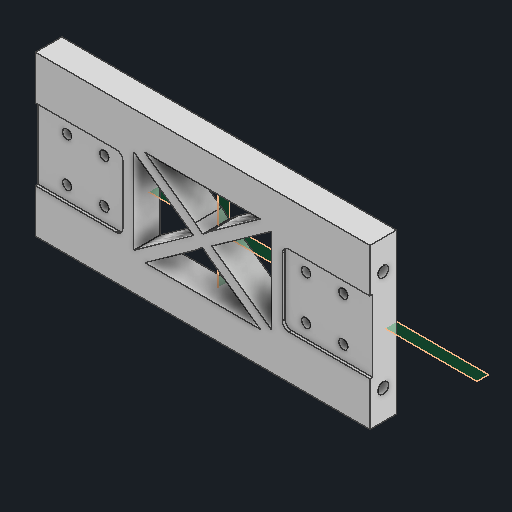
# Autodesk Inventor part: Part1
Saved by Autodesk Inventor 2026 (Build 300175000, 175)
## iProperties
Created: 2026-08-13
Part Number: Part1
Material: Generic
Document SubType Name: Modeling
Designer: imcle
Density: 1 g/cm^3
Appearance: Default
Author: imcle
Autodesk Inventor part; units mm, degrees
ref_plane "YZ Plane" through (0, 0, 0) normal (1, 0, 0) x (0, 1, 0)
ref_plane "XZ Plane" through (0, 0, 0) normal (0, 1, 0) x (-1, 0, 0)
ref_plane "XY Plane" through (0, 0, 0) normal (0, 0, 1) x (1, 0, 0)
sketch "Sketch1" plane through (0, 0, 0) normal (0, 0, 1) x (1, 0, 0)
  line L0 (0, 0) -> (120, 0)
  line L1 (120, 0) -> (120, 50)
  line L2 (120, 50) -> (0, 50)
  line L3 (0, 50) -> (0, 0)
  dimension "d0" = 120
  dimension "d1" = 50
  constraints: 8 end point, 2 parallel, 1 horizontal, 1 perpendicular
  measures "d0" distance of L2.end L1.end
  measures "d1" distance of L1.end L0.end
extrude "Extrusion1" add sketch "Sketch1" along normal blind 10
sketch "Sketch2" plane through (0, 0, 10) normal (0, 0, 1) x (1, 0, 0)
  line L0 (0, 50) -> (0, 0) projected
  line L1 (0, 11.5) -> (0, 38.5)
  line L2 (0, 38.5) -> (27.5, 38.5)
  line L3 (30, 36) -> (30, 14)
  line L4 (27.5, 11.5) -> (0, 11.5)
  line L5 (0, 11.5) -> (0, 38.5)
  arc A0 (30, 36) -> (27.5, 38.5) centre (27.5, 36) ccw
  arc A1 (27.5, 11.5) -> (30, 14) centre (27.5, 14) ccw
  point P0 (0, 25)
  point P1 (30, 11.5)
  point P2 (30, 38.5)
  dimension "d4" = 27
  dimension "d5" = 30
  dimension "d8" = 2.5
  dimension "d9" = 2.5
  constraints: 10 end point, 5 point on line, 4 point on circle, 4 tangent, 2 centre point, 2 midpoint, 2 parallel, 1 horizontal, 1 perpendicular
  measures "d4" distance of L1.start L1.end
  measures "d5" distance of point (30, 11.5) L4.end
  measures "d8" radius of A0
  measures "d9" radius of A1
extrude "Extrusion2" cut sketch "Sketch2" against normal blind 1
sketch "Sketch3" plane through (0, 0, 9) normal (0, 0, 1) x (1, 0, 0)
  arc A0 (30, 36) -> (27.5, 38.5) centre (27.5, 36) ccw projected
  line L0 (0, 38.5) -> (27.5, 38.5) projected
  line L1 (0, 38.5) -> (27.5, 38.5) projected
  line L2 (0, 11.5) -> (0, 38.5) projected
  line L3 (27.5, 11.5) -> (0, 11.5) projected
  arc A1 (27.5, 11.5) -> (30, 14) centre (27.5, 14) ccw projected
  line L4 (30, 36) -> (30, 14) projected
  arc A2 (30, 36) -> (27.5, 38.5) centre (27.5, 36) ccw projected
  line L5 (30, 36) -> (30, 14) projected
  line L6 (30, 38.5) -> (22, 38.5)
  line L7 (22, 38.5) -> (22, 33.25)
  line L8 (22, 33.25) -> (30, 33.25)
  line L9 (30, 33.25) -> (30, 38.5)
  circle A3 centre (22, 33.25) radius 1.75
  line L10 (30, 38.5) -> (8, 38.5)
  line L11 (8, 38.5) -> (8, 33.25)
  line L12 (8, 33.25) -> (30, 33.25)
  line L13 (30, 33.25) -> (30, 38.5)
  circle A4 centre (8, 33.25) radius 1.75
  line L14 (30, 25) -> (16.651, 25)
  circle A5 centre (22, 16.75) radius 1.75
  circle A6 centre (8, 16.75) radius 1.75
  point P0 (0, 0)
  dimension "d10" = 8
  dimension "d11" = 5.25
  dimension "d12" = 3.5
  dimension "d13" = 22
  dimension "d14" = 3.5
  constraints: 18 end point, 4 centre point, 4 parallel, 3 horizontal, 2 coincident, 2 perpendicular, 2 symmetric about line, 1 midpoint, 2 other
  measures "d10" distance of L8.end L7.end
  measures "d11" distance of L7.end L6.end
  measures "d12" diameter of A3
  measures "d13" distance of L12.end L11.end
  measures "d14" diameter of A4
extrude "Extrusion3" cut sketch "Sketch3" against normal up to surface (9 mm away) contours A3 L12 L8 | L8 L7 A3 | L7 L12 A3 | A4 L12 L11 | L11 L12 A4 | A5 | A6
ref_plane "Work Plane1" through (60, 0, 0) normal (-1, 0, 0) x (0, 0, 1)
mirror "Mirror1" about plane through (60, 0, 0) normal (-1, 0, 0) of "Extrusion2", "Extrusion3"
ref_plane "Work Plane2" through (0, 25, 0) normal (0, -1, 0) x (1, 0, 0)
sketch "Sketch6" plane through (0, 0, 0) normal (-1, 0, 0) x (0, 0, 1)
  line L0 (9, 38.5) -> (10, 38.5) projected
  line L1 (9, 11.5) -> (9, 38.5) projected
  line L2 (10, 11.5) -> (9, 11.5) projected
  line L3 (0, 50) -> (0, 0) projected
  line L4 (0, 0) -> (10, 0) projected
  line L5 (10, 11.5) -> (10, 0) projected
  line L6 (0, 50) -> (10, 50) projected
  line L7 (10, 50) -> (10, 38.5) projected
extrude "Extrusion6" add sketch "Sketch6" along normal blind 3
mirror "Mirror4" about plane through (60, 0, 0) normal (-1, 0, 0) of "Extrusion6"
sketch "Sketch7" plane through (0, 0, 0) normal (0, 0, -1) x (-1, 0, 0)
  circle A0 centre (-112, 16.75) radius 1.75 projected
  circle A1 centre (-112, 16.75) radius 3.25
  point P0 (0, 0)
  dimension "d27" = 6.5
  constraints: 1 centre point, 1 coincident
  measures "d27" diameter of A1
extrude "Extrusion7" cut sketch "Sketch7" against normal blind 4
pattern_linear "Rectangular Pattern1" count 2 spacing -14 along (1, 0, 0) count 2 spacing 16.5 along (0, 1, 0) of "Extrusion7"
mirror "Mirror5" about plane through (60, 0, 0) normal (-1, 0, 0) of "Extrusion7", "Rectangular Pattern1"
sketch "Sketch9" plane through (-3, 0, 0) normal (-1, 0, 0) x (0, 0, 1)
  line L0 (10, 50) -> (5, 50)
  line L1 (5, 50) -> (5, 44)
  line L2 (5, 44) -> (10, 44)
  line L3 (10, 44) -> (10, 50)
  circle A0 centre (5, 44) radius 2.05
  point P0 (0, 0)
  dimension "d36" = 5
  dimension "d37" = 6
  dimension "d38" = 4.1
  constraints: 8 end point, 2 parallel, 1 centre point, 1 coincident, 1 horizontal, 1 perpendicular
  measures "d36" distance of L2.end L1.end
  measures "d37" distance of L1.end L0.end
  measures "d38" diameter of A0
extrude "Extrusion8" cut sketch "Sketch9" against normal blind 5.5 contours A0 L2 L1 | L1 L2 A0
mirror "Mirror6" about plane through (0, 25, 0) normal (0, -1, 0) of "Extrusion8"
sketch "Sketch12" plane through (0, 0, 0) normal (0, 0, -1) x (-1, 0, 0)
  line L0 (-123, 0) -> (3, 0) projected
  line L1 (-60, 0) -> (-60, 50)
  line L2 (3, 50) -> (-123, 50) projected
  line L3 (-88, 5) -> (-88, 45)
  line L4 (-88, 45) -> (-32, 45)
  line L5 (-32, 45) -> (-32, 5)
  line L6 (-32, 5) -> (-88, 5)
  line L7 (-88, 5) -> (-32, 45) construction
  line L8 (-88, 45) -> (-32, 5) construction
  line L9 (-60, 45) -> (-60, 43)
  line L10 (-63.9713, 27.8366) -> (-62.8088, 29.4641)
  line L11 (-62.8088, 29.4641) -> (-85.7421, 45.845)
  line L12 (-63.8051, 43) -> (-81.7591, 43)
  line L13 (-60, 43) -> (-60, 27.1502)
  line L14 (-62.8088, 29.4641) -> (-60, 27.1502)
  line L15 (-88, 25) -> (-86, 25)
  line L16 (-86, 25) -> (-86, 27)
  line L17 (-79.67, 39.05) -> (-80.8325, 37.4226)
  line L18 (-80.8325, 37.4226) -> (-69.7179, 29.4835)
  line L19 (-86, 41.1136) -> (-86, 27)
  line L20 (-86, 41.1136) -> (-80.8325, 37.4226)
  line L21 (-69.7179, 29.4835) -> (-63.4409, 25)
  line L22 (-63.4409, 25) -> (-86, 25)
  line L23 (-63.8051, 43) -> (-60, 43)
  line L24 (-57.1912, 29.4641) -> (-34.2579, 45.845)
  line L25 (-56.1949, 43) -> (-38.2409, 43)
  line L26 (-57.1912, 29.4641) -> (-60, 27.1502)
  line L27 (-34, 25) -> (-34, 27)
  line L28 (-39.1675, 37.4226) -> (-50.2821, 29.4835)
  line L29 (-34, 41.1136) -> (-34, 27)
  line L30 (-34, 41.1136) -> (-39.1675, 37.4226)
  line L31 (-50.2821, 29.4835) -> (-56.5591, 25)
  line L32 (-56.5591, 25) -> (-34, 25)
  line L33 (-56.1949, 43) -> (-60, 43)
  line L34 (-88, 5) -> (-32, 45) construction
  line L35 (-62.8088, 20.5359) -> (-85.7421, 4.155)
  line L36 (-63.8051, 7) -> (-81.7591, 7)
  line L37 (-62.8088, 20.5359) -> (-60, 22.8498)
  line L38 (-86, 25) -> (-86, 23)
  line L39 (-80.8325, 12.5774) -> (-69.7179, 20.5165)
  line L40 (-86, 8.8864) -> (-86, 23)
  line L41 (-86, 8.8864) -> (-80.8325, 12.5774)
  line L42 (-69.7179, 20.5165) -> (-63.4409, 25)
  line L43 (-34, 25) -> (-34, 23)
  line L44 (-34, 8.8864) -> (-34, 23)
  line L45 (-34, 8.8864) -> (-39.1675, 12.5774)
  line L46 (-39.1675, 12.5774) -> (-50.2821, 20.5165)
  line L47 (-50.2821, 20.5165) -> (-56.5591, 25)
  line L48 (-57.1912, 20.5359) -> (-34.2579, 4.155)
  line L49 (-56.1949, 7) -> (-38.2409, 7)
  line L50 (-56.1949, 7) -> (-60, 7)
  line L51 (-57.1912, 20.5359) -> (-60, 22.8498)
  line L52 (-60, 7) -> (-63.8051, 7)
  point P0 (0, 0)
  point P1 (-60, 25)
  dimension "d41" = 40
  dimension "d42" = 56
  dimension "d43" = 2
  dimension "d45" = 2
  dimension "d46" = 2
  dimension "d47" = 2
  dimension "d48" = 2
  constraints: 102 end point, 28 symmetric about line, 12 point on line, 7 midpoint, 6 parallel, 6 perpendicular, 2 horizontal, 1 vertical
  measures "d41" distance of L3.start L3.end
  measures "d42" distance of L3.end L4.end
  measures "d43" distance of L9.start L9.end
  measures "d45" distance of L10.start L10.end
  measures "d46" distance of L15.start L15.end
  measures "d47" distance of L15.end L16.end
  measures "d48" distance of L17.start L17.end
extrude "Extrusion9" cut sketch "Sketch12" against normal up to surface (10 mm away) contours L52 L36 L35 L37 L1 | L1 L51 L48 L49 L50 | L14 L11 L12 L23 L1 | L1 L33 L25 L24 L26 | L16 L19 L20 L18 L21 L22 | L22 L42 L39 L41 L40 L38 | L32 L31 L28 L30 L29 L27 | L43 L44 L45 L46 L47 L32
sketch "Sketch13" plane through (-3, 50, 10) normal (0, 1, 0) x (1, 0, 0)
  line L0 (126, 0) -> (126, 10) projected
  line L1 (0, 10) -> (126, 10) projected
  line L2 (0, 0) -> (126, 0) projected
  line L3 (0, 0) -> (0, 10) projected
  point P0 (3, 10)
extrude "Extrusion10" add sketch "Sketch13" along normal blind 5
mirror "Mirror7" about plane through (0, 25, 0) normal (0, -1, 0) of "Extrusion10"
mirror "Mirror8" about plane through (60, 0, 0) normal (-1, 0, 0) of "Extrusion8", "Mirror6"
body "Solid1"
